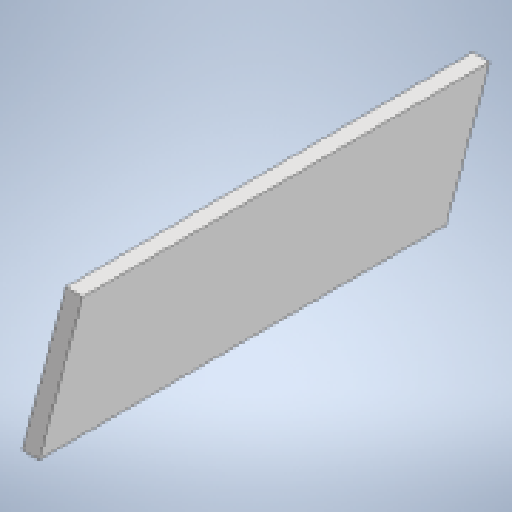
# Autodesk Inventor part: noz2
Saved by Autodesk Inventor 2023 (Build 270158000, 158)
## iProperties
Created: 2023-12-19
Part Number: noz2
Material: Ogólny
Document SubType Name: Modeling
Designer: Kamil
Density: 1 g/cm^3
Appearance: Domyślna
Author: Kamil
Autodesk Inventor part; units mm, degrees
ref_plane "YZ Plane" through (0, 0, 0) normal (1, 0, 0) x (0, 1, 0)
ref_plane "XZ Plane" through (0, 0, 0) normal (0, 1, 0) x (-1, 0, 0)
ref_plane "XY Plane" through (0, 0, 0) normal (0, 0, 1) x (1, 0, 0)
sketch "Szkic1" plane through (0, 0, 0) normal (0, 0, 1) x (1, 0, 0)
  line L0 (-10.5, 0) -> (0, 0) projected
  line L1 (0, 2) -> (-10.5, 2)
  line L2 (0, 2) -> (-5.359, -18)
  line L3 (-3.8837, -4.7669) -> (-2.0706, 2)
  line L4 (-3.8837, -4.7669) -> (-7.4295, -18)
  line L5 (-7.4295, -18) -> (-5.359, -18)
  dimension "d0" = 2
  dimension "d1" = 75
  dimension "d3" = 2
  dimension "d4" = 20
  constraints: 10 end point, 2 horizontal, 2 parallel, 1 point on line, 1 vertical alignment
  measures "d0" distance between parallel lines of L1 L0
  measures "d1" angle of L1 L2
  measures "d3" distance between parallel lines of L3 L2
  measures "d4" distance between parallel lines of L1 L5
extrude "Wyciągnięcie proste1" add sketch "Szkic1" against normal blind 50
